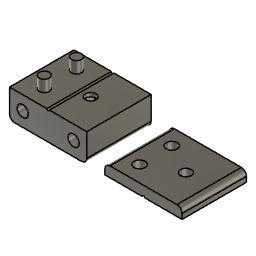
single chanel puller (rubber band) (Autodesk Fusion 360 design; units mm, degrees)
Autodesk Fusion 360 part; units mm, degrees
sketch "Sketch1" plane through (0, 0, 0) normal (0, 0, 1) x (1, 0, 0) in component "bottom bit"
  line L0 (0, 0) -> (30, 0)
  line L1 (30, 0) -> (30, 25)
  line L2 (30, 25) -> (0, 25)
  line L3 (0, 25) -> (0, 0)
  dimension "d1" = 30
  dimension "d2" = 25
  constraint horizontal L0
  constraint vertical L1
  constraint horizontal L2
  constraint vertical L3
  constraint coincident L0.start L3.end
  measures "d1" distance of L0.start L0.end
  measures "d2" distance of L0.start L2.end
extrude "Extrude1" add sketch "Sketch1" along normal blind 11 makes body 1 in component "bottom bit"
sketch "Sketch2" plane through (0, 0, 0) normal (0, -1, 0) x (1, 0, 0) in component "bottom bit"
  line L0 (0, 0) -> (30, 0)
  line L1 (30, 0) -> (30, 11)
  line L2 (30, 11) -> (0, 11)
  line L3 (0, 11) -> (0, 0)
  line L4 (0, 11) -> (30, 0) construction
  line L5 (30, 11) -> (0, 0) construction
  line L6 (0, 5.5) -> (30, 5.5) construction
  line L7 (15, 11) -> (15, 0) construction
  line L8 (15, 11) -> (0, 0) construction
  line L9 (0, 11) -> (15, 0) construction
  line L10 (7.5876, 11) -> (7.5876, 0) construction
  line L11 (0, 5.5) -> (5.125, 5.5) construction
  circle A0 centre (5.125, 5.5) radius 2.1875
  line L12 (5.125, 5.5) -> (2.9375, 5.5) construction
  circle A1 centre (24.875, 5.5) radius 2.1875
  dimension "d5" = 5.125
  dimension "d6" = 4.375
  dimension "d7" = 2.9375
  dimension "d37" = 4.375
  constraint coincident L2.end L3.start
  constraint coincident L0.end L1.start
  constraint coincident L1.end L2.start
  constraint coincident L0.start L3.end
  constraint midpoint L3 L6.start
  constraint midpoint L1 L6.end
  constraint midpoint L2 L7.start
  constraint midpoint L0 L7.end
  constraint coincident L2 L10.start
  constraint perpendicular L6 L10
  constraint perpendicular L3 L11
  constraint coincident L11.end A0.centre
  constraint coincident L11 L12.end
  constraint coincident A0 L12.end
  constraint symmetric L7 A0 A1
  measures "d5" distance of L6.start L11.end
  measures "d6" diameter of A0
  measures "d7" distance of L6.start L12.end
  measures "d37" diameter of A1
extrude "Extrude2" cut sketch "Sketch2" against normal blind 40 contours A0 | A1 bodies 1 in component "bottom bit"
sketch "Sketch3" plane through (0, 0, 0) normal (0, -1, 0) x (1, 0, 0) in component "bottom bit"
  circle A0 centre (24.875, 5.5) radius 2.1875
  circle A1 centre (5.125, 5.5) radius 2.1875
  line L0 (0, 0) -> (30, 0)
  line L1 (30, 0) -> (30, 11)
  line L2 (30, 11) -> (0, 11)
  line L3 (0, 11) -> (0, 0)
  circle A2 centre (15, 11) radius 0.5
  dimension "d10" = 1
  constraint midpoint L2 A2.centre
  measures "d10" diameter of A2
extrude "Extrude3" cut sketch "Sketch3" against normal blind 30 contours L2 A2 picked at (14.8961, 10.7714) bodies 1 in component "bottom bit"
sketch "Sketch4" plane through (0, 0, 11) normal (0, 0, 1) x (-1, 0, 0) in component "bottom bit"
  line L0 (-14.5, 0) -> (-14.5, -25)
  line L1 (-14.5, -25) -> (0, -25)
  line L2 (0, -25) -> (0, 0)
  line L3 (0, 0) -> (-14.5, 0)
  line L4 (0, -25) -> (-14.5, 0) construction
  line L5 (-14.5, -25) -> (0, 0) construction
  line L6 (-7.25, -12.5) -> (0, -12.5) construction
  line L7 (-7.25, -12.5) -> (-14.5, -12.5) construction
  line L8 (0, -25) -> (-14.5, -12.5) construction
  line L9 (0, -12.5) -> (-14.5, -25) construction
  circle A0 centre (-7.25, -18.75) radius 1.95
  circle A1 centre (-7.25, -6.25) radius 1.95
  dimension "d13" = 3.9
  constraint coincident L1.end L2.start
  constraint coincident L0.start L3.end
  constraint coincident L0.end L1.start
  constraint coincident L2.end L3.start
  constraint midpoint L5 L6.start
  constraint midpoint L2 L6.end
  constraint midpoint L0 L7.end
  constraint midpoint L8 A0.centre
  constraint symmetric L7 A0 A1
  measures "d13" diameter of A0
extrude "Extrude4" add sketch "Sketch4" along normal blind 4.5 contours A0 | A1 bodies 1 in component "bottom bit"
sketch "Sketch5" plane through (0, 0, 11) normal (0, 0, 1) x (-1, 0, 0) in component "bottom bit"
  line L0 (-15.5, -25) -> (-15.5, 0)
  line L1 (-15.5, 0) -> (-30, 0)
  line L2 (-30, 0) -> (-30, -25)
  line L3 (-30, -25) -> (-15.5, -25)
  line L4 (-15.5, -25) -> (-30, 0) construction
  line L5 (-30, -25) -> (-15.5, 0) construction
  circle A0 centre (-19, -12.5) radius 2.05
  dimension "d16" = 4.1
  dimension "d36" = 3.5
  constraint coincident L0.start L3.end
  constraint coincident L1.end L2.start
  constraint coincident L2.end L3.start
  constraint coincident L0.end L1.start
  measures "d16" diameter of A0
  measures "d36" distance of L0 A0.centre
extrude "Extrude5" cut sketch "Sketch5" against normal blind 11 contours A0 bodies 1 in component "bottom bit"
ref_plane "WorkPlane1" through (7.25, 12.5, 21) normal (0, 0, 1) x (1, 0, 0) in component "top bit"
sketch "Sketch1 (2)" plane through (0, 0, 21) normal (0, 0, 1) x (1, 0, 0) in component "top bit"
  line L0 (0, 0) -> (30, 0)
  line L1 (30, 0) -> (30, 25)
  line L2 (30, 25) -> (0, 25)
  line L3 (0, 25) -> (0, 0)
  constraint horizontal L0
  constraint vertical L1
  constraint horizontal L2
  constraint vertical L3
  constraint coincident L0.start L3.end
extrude "Extrude1'" add sketch "Sketch1 (2)" along normal blind 4 separate body makes body 2 in component "top bit"
sketch "Sketch2 (2)" plane through (0, 0, 25) normal (0, 0, 1) x (-1, 0, 0) in component "top bit"
  line L0 (0, -25) -> (0, 0)
  line L1 (0, 0) -> (-30, 0)
  line L2 (-30, 0) -> (-30, -25)
  line L3 (-30, -25) -> (0, -25)
  circle A0 centre (-19, -12.5) radius 2.05
  circle A1 centre (-7.25, -18.75) radius 1.95
  circle A2 centre (-7.25, -6.25) radius 1.95
  circle A3 centre (-19, -12.5) radius 2.05
  circle A4 centre (-7.25, -18.75) radius 2.125
  circle A5 centre (-7.25, -6.25) radius 2.125
  point P0 (-9.2, -6.25)
  dimension "d22" = 4.25
  dimension "d23" = 4.25
  constraint concentric A0 A3
  constraint concentric A1 A4
  constraint concentric A2 A5
  measures "d22" diameter of A4
  measures "d23" diameter of A5
extrude "Extrude2'" cut sketch "Sketch2 (2)" against normal blind 8 contours A0 A3 | A1 | A2 | A4 | A5 bodies 2 in component "top bit"
sketch "Sketch3 (2)" plane through (0, 0, 0) normal (0, -1, 0) x (1, 0, 0) in component "top bit"
  line L0 (0, 21) -> (30, 21)
  line L1 (30, 21) -> (30, 25)
  line L2 (30, 25) -> (0, 25)
  line L3 (0, 25) -> (0, 21)
  circle A0 centre (15, 21) radius 0.5
  dimension "d26" = 1
  constraint midpoint L0 A0.centre
  measures "d26" diameter of A0
extrude "Extrude3'" cut sketch "Sketch3 (2)" against normal blind 100 contours L0 A0 picked at (15.1222, 21.2116) bodies 2 in component "top bit"
sketch "Sketch6" plane through (0, 0, 0) normal (0, 0, -1) x (1, 0, 0) in component "bottom bit"
  circle A0 centre (19, -12.5) radius 2.05
  line L0 (0, 0) -> (0, -25)
  line L1 (0, -25) -> (30, -25)
  line L2 (30, -25) -> (30, 0)
  line L3 (30, 0) -> (0, 0)
  line L4 (21.15, -16.2239) -> (23.3, -12.5)
  line L5 (23.3, -12.5) -> (21.15, -8.7761)
  line L6 (21.15, -8.7761) -> (16.85, -8.7761)
  line L7 (16.85, -8.7761) -> (14.7, -12.5)
  line L8 (14.7, -12.5) -> (16.85, -16.2239)
  line L9 (16.85, -16.2239) -> (21.15, -16.2239)
  point P0 (19, -12.5)
  dimension "d29" = 4.3
  constraint coincident P0 A0.centre
  constraint parallel L1 L9
  measures "d29" distance of L4.start P0
extrude "Extrude6" cut sketch "Sketch6" against normal blind 9.5 contours L4 L5 L6 L7 L8 L9 bodies 1 in component "bottom bit"
fillet "Fillet1" radius 2 2 edges at (30, 12.5, 25) (0, 12.5, 25) on bodies 2 in component "top bit"
fillet "Fillet1'" radius 2 2 edges at (30, 12.5, 0) (0, 12.5, 0) on bodies 1 in component "bottom bit"
move_body "Move1" bodies 2 to x (1, 0, 0) y (0, 1, 0) z (0, 0, 1) at (37, 0, -21) in component "top bit"
component "bottom bit" placed x (1, 0, 0) y (0, 1, 0) z (0, 0, 1) at (0, 0, 0)
component "top bit" placed x (1, 0, 0) y (0, 1, 0) z (0, 0, 1) at (0, 0, 0) in component "bottom bit"
